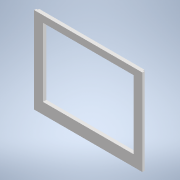
# Autodesk Inventor part: Arcade_Front
Saved by Autodesk Inventor 2022 (Build 260153000, 153)
## iProperties
Created: 2023-12-22
Part Number: Arcade_Front
Material: Generic
Document SubType Name: Modeling
Designer: Petr Černý
Density: 1 g/cm^3
Appearance: Default
Author: Petr Černý
Autodesk Inventor part; units mm, degrees
ref_plane "YZ Plane" through (0, 0, 0) normal (1, 0, 0) x (0, 1, 0)
ref_plane "XZ Plane" through (0, 0, 0) normal (0, 1, 0) x (-1, 0, 0)
ref_plane "XY Plane" through (0, 0, 0) normal (0, 0, 1) x (1, 0, 0)
sketch "Sketch1" plane through (0, 0, 0) normal (0, 0, 1) x (1, 0, 0)
  line L0 (-208.5912, 171.4818) -> (201.4088, 171.4818)
  line L1 (201.4088, 171.4818) -> (201.4088, -138.5182)
  line L2 (201.4088, -138.5182) -> (-208.5912, -138.5182)
  line L3 (-208.5912, -138.5182) -> (-208.5912, 171.4818)
  line L4 (-248.5912, 201.4818) -> (241.4088, 201.4818)
  line L5 (241.4088, 201.4818) -> (241.4088, -188.5182)
  line L6 (241.4088, -188.5182) -> (-248.5912, -188.5182)
  line L7 (-248.5912, -188.5182) -> (-248.5912, 201.4818)
  point P0 (0, 0)
  dimension "d0" = 410
  dimension "d1" = 310
  dimension "d2" = 490
  dimension "d3" = 40
  dimension "d4" = 390
  dimension "d5" = 50
  constraints: 16 end point, 4 parallel, 2 horizontal, 2 perpendicular
  measures "d0" distance of L0.start L0.end
  measures "d1" distance of L0.end L1.end
  measures "d2" distance of L4.start L4.end
  measures "d3" distance between parallel lines of L7 L3
  measures "d4" distance between parallel lines of L6 L4
  measures "d5" distance between parallel lines of L2 L6
extrude "Extrusion1" add sketch "Sketch1" along normal blind 15
sketch "Sketch2" plane through (241.4088, -188.5182, 0) normal (1, 0, 0) x (0, 0, -1)
  line L0 (0, 390) -> (-15, 390) projected
  line L1 (0, 390) -> (-5, 390)
  line L2 (-5, 390) -> (-5, 0)
  line L3 (-5, 0) -> (0, 0)
  line L4 (0, 0) -> (0, 390)
  point P0 (0, 188.5182)
  dimension "d8" = 5
  dimension "d9" = 390
  constraints: 8 end point, 2 parallel, 1 horizontal, 1 perpendicular
  measures "d8" distance of L3.end L2.end
  measures "d9" distance of L2.end L1.end
extrude "Extrusion2" cut sketch "Sketch2" against normal blind 7
sketch "Sketch3" plane through (-248.5912, -188.5182, 0) normal (-1, 0, 0) x (0, 0, 1)
  line L0 (0, 390) -> (0, 0) projected
  line L1 (5, 0) -> (5, 390) projected
  line L2 (0, 390) -> (5, 390)
  line L3 (5, 390) -> (5, 0)
  line L4 (5, 0) -> (0, 0)
  line L5 (0, 0) -> (0, 390)
  point P0 (0, 188.5182)
  point P1 (0, 0)
  dimension "d12" = 5
  dimension "d13" = 390
  constraints: 8 end point, 2 parallel, 1 horizontal, 1 perpendicular
  measures "d12" distance of L1.start L4.end
  measures "d13" distance of L2.end L1.start
extrude "Extrusion3" cut sketch "Sketch3" against normal blind 7
sketch "Sketch4" plane through (0, 0, 0) normal (0, 0, -1) x (-1, 0, 0)
  line L0 (-234.4088, 201.4818) -> (241.5912, 201.4818) projected
  line L1 (-234.4088, 201.4818) -> (241.5912, 201.4818)
  line L2 (241.5912, 201.4818) -> (241.5912, -188.5182)
  line L3 (241.5912, -188.5182) -> (-234.4088, -188.5182)
  line L4 (-234.4088, -188.5182) -> (-234.4088, 201.4818)
  line L5 (208.5912, 171.4818) -> (-201.4088, 171.4818) projected
  line L6 (-201.4088, 171.4818) -> (208.5912, 171.4818)
  line L7 (208.5912, 171.4818) -> (208.5912, -138.5182)
  line L8 (208.5912, -138.5182) -> (-201.4088, -138.5182)
  line L9 (-201.4088, -138.5182) -> (-201.4088, 171.4818)
  point P0 (0, 0)
  constraints: 16 end point, 4 parallel, 2 horizontal, 2 perpendicular
extrude "Extrusion4" add sketch "Sketch4" along normal blind 1
body "Solid1"
